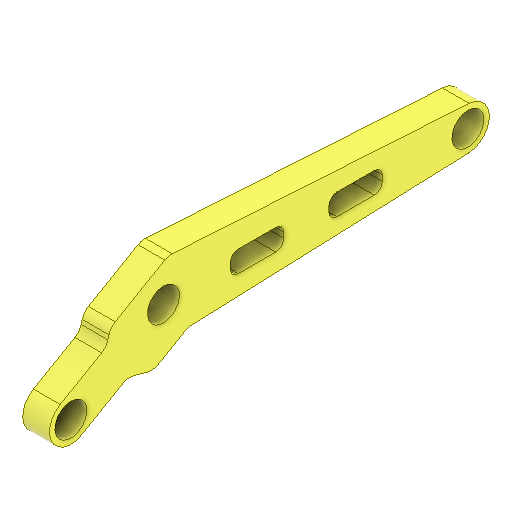
# Autodesk Inventor part: Link_ECH
Saved by Autodesk Inventor 2026.2 (Build 302298000, 298)
## iProperties
Created: 2025-12-27
Part Number: Link_ECH
Material: ABS 塑膠
Document SubType Name: Modeling
Designer: Hsiangyu
Density: 1.06 g/cm^3
Appearance: 平滑 - 黃色
Author: Hsiangyu
Autodesk Inventor part; units mm, degrees
ref_plane "YZ Plane" through (0, 0, 0) normal (1, 0, 0) x (0, 1, 0)
ref_plane "XZ Plane" through (0, 0, 0) normal (0, 1, 0) x (-1, 0, 0)
ref_plane "XY Plane" through (0, 0, 0) normal (0, 0, 1) x (1, 0, 0)
sketch "草圖1" plane through (0, 0, 0) normal (1, 0, 0) x (0, 1, 0)
  line L0 (0, 0) -> (0, -113.9)
  line L1 (0, 0) -> (-20, 34.641)
  circle A0 centre (0, 0) radius 6
  circle A1 centre (0, 0) radius 8
  circle A2 centre (-20, 34.641) radius 6
  circle A3 centre (-20, 34.641) radius 8
  circle A4 centre (0, -113.9) radius 6
  circle A5 centre (0, -113.9) radius 8
  line L2 (-13.0718, 38.641) -> (-3.0718, 21.3205)
  line L3 (-3.0718, 21.3205) -> (2.3923, 19.8564)
  line L4 (2.3923, 19.8564) -> (14.8923, -1.7942)
  line L5 (14.8923, -1.7942) -> (7.985, -114.3898)
  line L6 (-26.9282, 30.641) -> (-16.9282, 13.3205)
  line L7 (-16.9282, 13.3205) -> (-19.4904, 3.7583)
  line L8 (-19.4904, 3.7583) -> (-11.9904, -9.2321)
  line L9 (-11.9904, -9.2321) -> (-7.9942, -114.2043)
  line L10 (4, -25) -> (-4, -25)
  line L11 (-4, -25) -> (-4, -45)
  line L12 (-4, -45) -> (4, -45)
  line L13 (4, -45) -> (4, -25)
  line L14 (4, -61.9) -> (-4, -61.9)
  line L15 (-4, -61.9) -> (-4, -81.9)
  line L16 (-4, -81.9) -> (4, -81.9)
  line L17 (4, -81.9) -> (4, -61.9)
  point P0 (0, -25)
  point P1 (0, -61.9)
  dimension "d0" = 113.9
  dimension "d1" = 40
  dimension "d2" = 150
  dimension "d3" = 12
  dimension "d4" = 16
  dimension "d5" = 12
  dimension "d6" = 16
  dimension "d7" = 12
  dimension "d8" = 16
  dimension "d9" = 25
  dimension "d10" = 15
  dimension "d11" = 135
  dimension "d12" = 135
  dimension "d13" = 20
  dimension "d14" = 20
  dimension "d15" = 15
  dimension "d16" = 12
  dimension "d21" = 20
  dimension "d22" = 8
  dimension "d23" = 25
  dimension "d25" = 32
  constraints: 36 end point, 8 parallel, 6 centre point, 6 coincident, 4 point on circle, 4 tangent, 2 equal length, 2 horizontal, 2 midpoint, 2 perpendicular, 2 vertical alignment, 1 vertical
  measures "d0" distance of L0.start L0.end
  measures "d1" distance of L0.start L1.end
  measures "d2" angle of L0 L1
  measures "d3" diameter of A0
  measures "d4" diameter of A1
  measures "d5" diameter of A4
  measures "d6" diameter of A5
  measures "d7" diameter of A2
  measures "d8" diameter of A3
  measures "d9" distance of L3.end L4.end
  measures "d10" distance of L7.end L8.end
  measures "d11" angle of L3 L4
  measures "d12" angle of L7 L8
  measures "d13" distance of L6.start L6.end
  measures "d14" distance of L2.start L2.end
  measures "d15" distance from line of A1.centre L8
  measures "d16" distance from line of A0.centre L4
  measures "d21" distance of L12.end L10.start
  measures "d22" distance of L11.end L12.end
  measures "d23" distance from line of L0.start L10
  measures "d25" distance from line of L0.end L16
extrude "擠出1" add sketch "草圖1" along normal blind 10 contours A0 L1 A1 L0 | L0 A1 L1 A0 | A1 L1 A3 L2 L3 L4 L5 A5 L0 L16 L17 L14 L12 L13 L10 | L0 L10 L11 L12 L14 L15 L16 A5 L9 L8 L7 L6 A3 L1 A1 | A3 | A5
fillet "圓角2" radius 3 8 edges at (5, 4, -45) (5, 4, -25) (5, -4, -25) (5, -4, -45) (5, -4, -61.9) (5, 4, -61.9) (5, -4, -81.9) (5, 4, -81.9)
fillet "圓角3" radius 5 6 edges at (5, 14.8923, -1.7942) (5, 2.3923, 19.8564) (5, -3.0718, 21.3205) (5, -16.9282, 13.3205) (5, -19.4904, 3.7583) (5, -11.9904, -9.2321)
equation "\"d5\" = d3"
equation "\"d6\" = d4"
equation "\"d7\" = d3"
equation "\"d8\" = d4"
equation "\"d12\" = d11"
equation "\"d14\" = d13"
